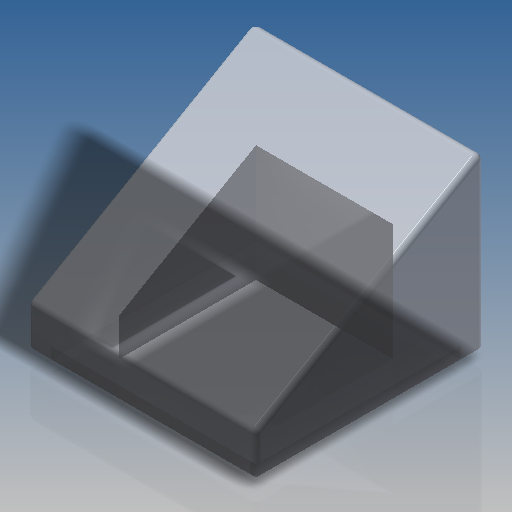
# Autodesk Inventor part: 54200-TransClear
Saved by Autodesk Inventor 2018.3 (Build 223284000, 284)
## iProperties
Created: 2014-06-03
Part Number: 54200-TransClear
Material: Polycarbonate
Document SubType Name: Modeling
Designer: D. Kohfeld
Density: 1.2 g/cm^3
Appearance: TransClear
Mass: 0.232769 g
Surface Area: 3.18183 cm^2
Volume: 0.193974 cm^3
Author: D. Kohfeld
Autodesk Inventor part; units mm, degrees
ref_plane "YZ Plane" through (0, 0, 0) normal (1, 0, 0) x (0, 1, 0)
ref_plane "XZ Plane" through (0, 0, 0) normal (0, 1, 0) x (-1, 0, 0)
ref_plane "XY Plane" through (0, 0, 0) normal (0, 0, 1) x (1, 0, 0)
sketch "Sketch10" plane through (0, 0, 0) normal (1, 0, 0) x (0, 1, 0)
  line L0 (0, 4) -> (1.7812, 4)
  line L1 (1.7812, 4) -> (6.4, -4)
  line L2 (6.4, -4) -> (0, -4)
  line L3 (0, -4) -> (0, 4)
  line L4 (0, 2.4) -> (1.32, 2.4)
  line L5 (1.32, 2.4) -> (4.0913, -2.4)
  line L6 (4.0913, -2.4) -> (0, -2.4)
  point P0 (0, 0)
  point P1 (0, 0)
  dimension "d91" = 8
  dimension "d92" = 6.4
  dimension "d103" = 30
  dimension "d109" = 1.32
  dimension "d110" = 1.6
  dimension "d111" = 1.6
  constraints: 14 end point, 3 horizontal, 2 parallel, 2 point on line, 1 coincident, 1 midpoint, 1 perpendicular
  measures "d91" distance of L2.end L0.start
  measures "d92" distance from line of L1.end L3
  measures "d103" angle of L1 L3
  measures "d109" distance from line of L4.end L3
  measures "d110" distance between parallel lines of L4 L0
  measures "d111" distance between parallel lines of L2 L6
extrude "Extrusion6" add sketch "Sketch10" along normal mid plane 8
sketch "Sketch11" plane through (-4, 0, -4) normal (0, -1, 0) x (1, 0, 0)
  line L0 (1.6, 6.4) -> (6.4, 6.4) construction
  line L1 (6.4, 6.4) -> (6.4, 1.6) construction
  line L2 (6.4, 1.6) -> (1.6, 1.6) construction
  line L3 (1.6, 1.6) -> (1.6, 6.4) construction
  circle A0 centre (4, 4) radius 2.4
  line L4 (8, 0) -> (0, 0) projected
  line L5 (8, 8) -> (8, 0) projected
  line L6 (0, 8) -> (8, 8) projected
  line L7 (0, 0) -> (0, 8) projected
  line L8 (0.4, 7.6) -> (7.6, 7.6)
  line L9 (7.6, 7.6) -> (7.6, 0.4)
  line L10 (7.6, 0.4) -> (0.4, 0.4)
  line L11 (0.4, 0.4) -> (0.4, 7.6)
  point P0 (0.4, 4)
  point P1 (4, 0.4)
  dimension "d96" = 4.8
  dimension "d104" = 0.4
  dimension "d105" = 0.4
  constraints: 16 end point, 4 parallel, 3 perpendicular, 3 tangent, 2 horizontal, 2 midpoint, 1 centre point, 1 coincident, 1 horizontal alignment, 1 vertical alignment
  measures "d96" diameter of A0
  measures "d104" distance between parallel lines of L6 L8
  measures "d105" distance between parallel lines of L7 L11
extrude "Extrusion9" cut sketch "Sketch10" along normal mid plane 4.8 contours L4 L5 L6 L3
extrude "Extrusion7" cut sketch "Sketch11" against normal blind 1.6 contours A0
extrude "Extrusion8" cut sketch "Sketch11" against normal blind 0.4 contours L4 L7 L6 L5
fillet "Fillet1" radius 0.2 8 edges at (-4, 4.0906, 0) (0, 1.7812, 4) (-4, 1.0906, 4) (4, 1.0906, 4) (4, 4.0906, 0) (4, 3.4, -4) (0, 6.4, -4) (-4, 3.4, -4)
equation "\"d91\" = lu"
equation "\"d92\" = 0.666667 * lh"
equation "\"d110\" = wall"
equation "\"d111\" = d110"
equation "\"d94\" = lu"
equation "\"d96\" = kd"
equation "\"d104\" = gw"
equation "\"d105\" = gw"
equation "\"d112\" = lu - 2 * wall"
equation "\"d97\" = 0.333333 * lh - topthk"
equation "\"d106\" = gh"
equation "\"d22\" = 2 * lf"
equation "\"lu\" = 8"
equation "\"lh\" = 9.6"
equation "\"wall\" = 1.6"
equation "\"kd\" = 4.8"
equation "\"gw\" = 0.4"
equation "\"topthk\" = 1.6"
equation "\"gh\" = 0.4"
equation "\"lf\" = 0.1"
body "Solid1"
body "Solid2"
